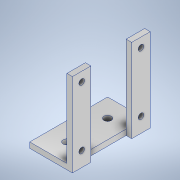
# Autodesk Inventor part: vertical_axis_motor_metal_holder
Saved by Autodesk Inventor 2021 (Build 250183000, 183)
## iProperties
Created: 2020-10-10
Part Number: vertical_axis_motor_metal_holder
Material: Aluminum 6061
Document SubType Name: Modeling
Designer: bober
Density: 2.7 g/cm^3
Appearance: Aluminum - Flat
Author: bober
Autodesk Inventor part; units mm, degrees
ref_plane "YZ Plane" through (0, 0, 0) normal (1, 0, 0) x (0, 1, 0)
ref_plane "XZ Plane" through (0, 0, 0) normal (0, 1, 0) x (-1, 0, 0)
ref_plane "XY Plane" through (0, 0, 0) normal (0, 0, 1) x (1, 0, 0)
sketch "Sketch1" plane through (0, 0, 0) normal (0, 1, 0) x (-1, 0, 0)
  line L0 (-10, 21) -> (10, 21)
  line L1 (10, 21) -> (10, -21)
  line L2 (10, -21) -> (-10, -21)
  line L3 (-10, -21) -> (-10, 21)
  line L4 (-10, 21) -> (10, -21) construction
  line L5 (10, 21) -> (-10, -21) construction
  point P0 (0, 0)
  dimension "d0" = 20
  dimension "d1" = 42
  constraints: 12 end point, 2 midpoint, 2 parallel, 1 horizontal, 1 perpendicular
  measures "d0" distance of L1.end L2.end
  measures "d1" distance of L0.end L1.end
extrude "Extrusion1" add sketch "Sketch1" along normal blind 3
sketch "Sketch2" plane through (10, 0, 21) normal (1, 0, 0) x (0, 0, -1)
  line L0 (0, 0) -> (10, 0)
  line L1 (10, 0) -> (10, 45)
  line L2 (10, 45) -> (0, 45)
  line L3 (0, 45) -> (0, 0)
  line L4 (42, 0) -> (0, 0) projected
  line L5 (42, 0) -> (32, 0)
  line L6 (32, 0) -> (32, 45)
  line L7 (32, 45) -> (42, 45)
  line L8 (42, 45) -> (42, 0)
  point P0 (21, 0)
  dimension "d4" = 10
  dimension "d5" = 45
  dimension "d6" = 10
  dimension "d7" = 45
  constraints: 16 end point, 4 parallel, 2 horizontal, 2 perpendicular
  measures "d4" distance of L2.end L1.end
  measures "d5" distance of L1.end L0.end
  measures "d6" distance of L6.end L7.end
  measures "d7" distance of L5.end L6.end
extrude "Extrusion2" add sketch "Sketch2" along normal blind 3
sketch "Sketch3" plane through (13, 0, 21) normal (1, 0, 0) x (0, 0, -1)
  circle A0 centre (5, 40) radius 1.5
  circle A1 centre (5, 8) radius 1.5
  point P0 (21, 0)
  dimension "d10" = 3
  dimension "d11" = 3
  constraints: 2 centre point
  measures "d10" diameter of A0
  measures "d11" diameter of A1
extrude "Extrusion3" cut sketch "Sketch3" against normal blind 3
mirror "Mirror1" about plane through (0, 0, 0) normal (0, 0, 1) of "Extrusion3"
sketch "Sketch5" plane through (0, 3, 0) normal (0, 1, 0) x (1, 0, 0)
  circle A0 centre (0, -11) radius 2
  circle A1 centre (0, 11) radius 2
  point P0 (0, 0)
  dimension "d18" = 4
  dimension "d19" = 4
  constraints: 2 centre point
  measures "d18" diameter of A0
  measures "d19" diameter of A1
extrude "Extrusion5" cut sketch "Sketch5" against normal blind 3
sketch "Sketch6" plane through (0, 3, 0) normal (0, 1, 0) x (1, 0, 0)
  point P0 (0, 0)
body "Solid1"
